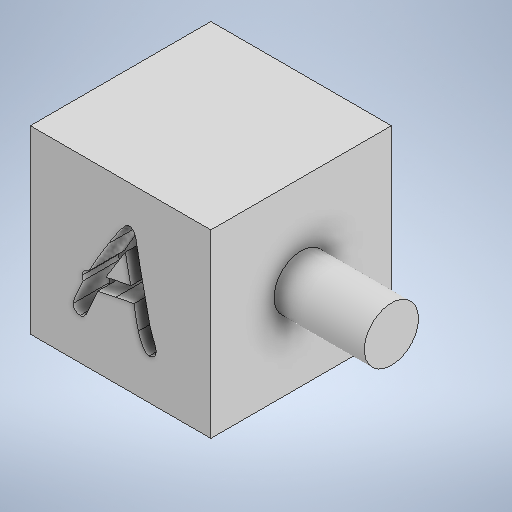
# Autodesk Inventor part: Adenosine
Saved by Autodesk Inventor 2025 (Build 290162000, 162)
## iProperties
Created: 2024-08-12
Part Number: Adenosine
Material: Generic
Document SubType Name: Modeling
Designer: kellst1
Density: 1 g/cm^3
Appearance: Default
Author: kellst1
Autodesk Inventor part; units mm, degrees
ref_plane "YZ Plane" through (0, 0, 0) normal (1, 0, 0) x (0, 1, 0)
ref_plane "XZ Plane" through (0, 0, 0) normal (0, 1, 0) x (-1, 0, 0)
ref_plane "XY Plane" through (0, 0, 0) normal (0, 0, 1) x (1, 0, 0)
sketch "Sketch1" plane through (0, 0, 0) normal (1, 0, 0) x (0, 1, 0)
  line L0 (0, 0) -> (10, 0)
  line L1 (10, 0) -> (10, -10)
  line L2 (10, -10) -> (0, -10)
  line L3 (0, -10) -> (0, 0)
  dimension "d0" = 10
  dimension "d1" = 10
  constraints: 8 end point, 2 parallel, 1 horizontal, 1 perpendicular
  measures "d0" distance of L1.end L2.end
  measures "d1" distance of L0.end L1.end
extrude "Extrusion1" add sketch "Sketch1" along normal blind 10
sketch "Sketch2" plane through (10, 0, 0) normal (1, 0, 0) x (0, 0, -1)
  circle A0 centre (5, 5) radius 1.5
  point P0 (0, 0)
  dimension "d4" = 3
  constraints: 1 centre point
  measures "d4" diameter of A0
extrude "Extrusion2" add sketch "Sketch2" along normal blind 5
sketch "Sketch4" plane through (0, 0, 0) normal (0, 0, 1) x (1, 0, 0)
  line L0 (1.8731, 7.9408) -> (4.4271, 7.9408) construction
  line L1 (4.4271, 7.9408) -> (4.4271, 4.8928) construction
  line L2 (4.4271, 4.8928) -> (1.8731, 4.8928) construction
  line L3 (1.8731, 4.8928) -> (1.8731, 7.9408) construction
  spline S0 degree 2 poles (6.5901, 2.2509) (6.243, 2.2509) (5.9854, 3.1396) knots 0 0 0 1 1 1
  spline S1 degree 2 poles (5.9854, 3.1396) (5.8854, 3.4814) (5.7382, 4.3281) knots 0 0 0 1 1 1
  spline S2 degree 2 poles (5.7382, 4.3281) (5.3543, 4.2755) (4.7338, 4.1388) knots 0 0 0 1 1 1
  line L4 (4.7338, 4.1388) -> (3.7347, 3.9337)
  spline S3 degree 2 poles (3.7347, 3.9337) (3.5454, 3.4394) (3.0826, 2.4876) knots 0 0 0 1 1 1
  spline S4 degree 2 poles (3.0826, 2.4876) (2.9617, 2.2772) (2.7566, 2.2772) knots 0 0 0 1 1 1
  spline S5 degree 2 poles (2.7566, 2.2772) (2.6041, 2.2772) (2.3674, 2.4981) (2.3674, 2.6558) knots 0 0 0 1 2 2 2
  spline S6 degree 2 poles (2.3674, 2.6558) (2.3674, 2.8399) (2.9354, 4.0336) knots 0 0 0 1 1 1
  spline S7 degree 2 poles (2.9354, 4.0336) (2.8723, 4.1335) (2.8723, 4.2597) knots 0 0 0 1 1 1
  spline S8 degree 2 poles (2.8723, 4.2597) (2.8723, 4.5647) (3.2404, 4.6541) knots 0 0 0 1 1 1
  spline S9 degree 2 poles (3.2404, 4.6541) (3.6716, 5.4587) (4.3289, 6.5104) knots 0 0 0 1 1 1
  spline S10 degree 2 poles (4.3289, 6.5104) (5.2229, 7.9408) (5.4437, 7.9408) knots 0 0 0 1 1 1
  spline S11 degree 2 poles (5.4437, 7.9408) (5.7382, 7.9408) (5.8486, 7.5253) knots 0 0 0 1 1 1
  line L5 (5.8486, 7.5253) -> (6.0853, 6.258)
  line L6 (6.0853, 6.258) -> (6.6479, 3.6339)
  line L7 (6.6479, 3.6339) -> (6.8636, 3.0397)
  spline S12 degree 2 poles (6.8636, 3.0397) (6.974, 2.7347) (6.974, 2.6296) knots 0 0 0 1 1 1
  spline S13 degree 2 poles (6.974, 2.6296) (6.974, 2.4718) (6.7426, 2.2509) (6.5901, 2.2509) knots 0 0 0 1 2 2 2
  line L8 (5.2597, 6.563) -> (4.1817, 4.8224)
  spline S14 degree 2 poles (4.1817, 4.8224) (4.6392, 4.9381) (5.5647, 5.1064) knots 0 0 0 1 1 1
  line L9 (5.5647, 5.1064) -> (5.2597, 6.563)
  point P0 (0, 0)
  constraints: 2 other
extrude "Extrusion4" cut sketch "Sketch4" against normal blind 2
body "Solid1"
